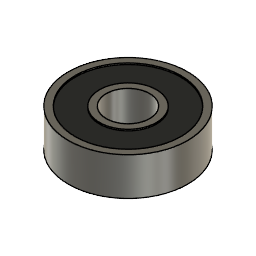
Bearing 608 (Autodesk Fusion 360 design; units mm, degrees)
Autodesk Fusion 360 part; units mm, degrees
sketch "Sketch1" plane through (0, 0, 0) normal (0, 0, 1) x (1, 0, 0)
  circle A0 centre (0, 0) radius 11
  circle A1 centre (0, 0) radius 9.75
  circle A2 centre (0, 0) radius 4
  circle A3 centre (0, 0) radius 5.25
  dimension "d1" = 22
  dimension "d2" = 19.5
  dimension "d3" = 8
  dimension "d4" = 10.5
  constraint coincident A0.centre A1.centre
  constraint concentric A0 A2
  constraint concentric A2 A3
  measures "d1" diameter of A0
  measures "d2" diameter of A1
  measures "d3" diameter of A2
  measures "d4" diameter of A3
extrude "Extrude1" add sketch "Sketch1" along normal blind 7 contours A0 makes body 1 in component "Outer Ring"
extrude "Extrude2" add sketch "Sketch1" along normal blind 6.5 from surface at 0.25 contours A1 bodies 1 in component "Outer Ring"
extrude "Extrude1'" add sketch "Sketch1" along normal blind 7 separate body contours A3 makes body 2 in component "Inner Ring"
component "Outer Ring" placed x (1, 0, 0) y (0, 1, 0) z (0, 0, 1) at (0, 0, 0)
component "Inner Ring" placed x (1, 0, 0) y (0, 1, 0) z (0, 0, 1) at (0, 0, 0)
